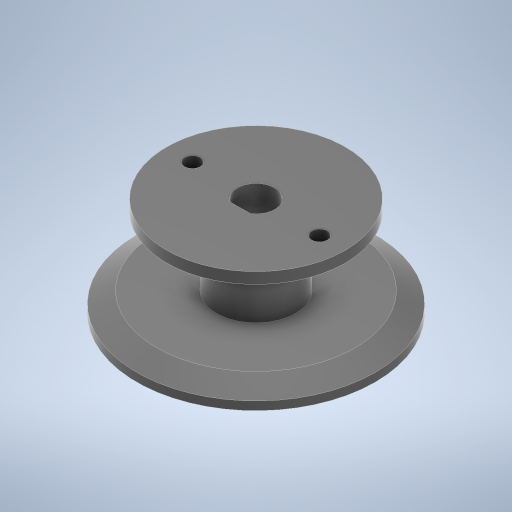
# Autodesk Inventor part: Pulley
Saved by Autodesk Inventor 2024 (Build 280153000, 153)
## iProperties
Created: 2023-12-18
Part Number: Pulley
Material: Generic
Document SubType Name: Modeling
Designer: greg
Density: 1 g/cm^3
Appearance: Smooth - Black
Author: greg
## iProperties of the stored document Pulley_3DPrint.ipt
Created: 2023-12-18
Part Number: Pulley_3DPrint
Material: Generic
Document SubType Name: Modeling
Designer: greg
Density: 1 g/cm^3
Appearance: Default
Author: greg
Autodesk Inventor part; units mm, degrees
ref_plane "YZ Plane" through (0, 0, 0) normal (1, 0, 0) x (0, 1, 0)
ref_plane "XZ Plane" through (0, 0, 0) normal (0, 1, 0) x (-1, 0, 0)
ref_plane "XY Plane" through (0, 0, 0) normal (0, 0, 1) x (1, 0, 0)
sketch "Sketch1" plane through (0, 0, 0) normal (0, 1, 0) x (-1, 0, 0)
  circle A0 centre (0, 0) radius 19.05
  dimension "d0" = 38.1
  constraints: 1 centre point, 1 coincident
  measures "d0" diameter of A0
extrude "Extrusion1" add sketch "Sketch1" along normal blind 3.175
sketch "Sketch2" plane through (0, 3.175, 0) normal (0, 1, 0) x (1, 0, 0)
  circle A0 centre (0, 0) radius 6.35
  dimension "d3" = 12.7
  constraints: 1 centre point, 1 coincident
  measures "d3" diameter of A0
extrude "Extrusion2" add sketch "Sketch2" along normal blind 6.35
sketch "Sketch3" plane through (0, 9.525, 0) normal (0, 1, 0) x (1, 0, 0)
  circle A0 centre (0, 0) radius 14.2875
  dimension "d6" = 28.575
  constraints: 1 centre point, 1 coincident
  measures "d6" diameter of A0
extrude "Extrusion3" add sketch "Sketch3" along normal blind 6.35
chamfer "Chamfer1" distance 7.9375 angle 30 1 edges at (-14.2875, 9.525, 0) measured on face at (-13.7875, 9.525, 0)
chamfer "Chamfer2" distance 3.175 angle 30 1 edges at (19.05, 3.175, 0) measured on face at (18.55, 3.175, 0)
sketch "Sketch4" plane through (0, 15.875, 0) normal (0, 1, 0) x (1, 0, 0)
  circle A0 centre (-10.16, 0) radius 1.27
  circle A1 centre (10.16, 0) radius 1.27
  circle A2 centre (0, 0) radius 6.35 projected
  dimension "d15" = 2.54
  dimension "d16" = 10.16
  dimension "d17" = 10.16
  constraints: 2 centre point, 1 equal radius
  measures "d15" diameter of A0
  measures "d16" distance of A0.centre A2.centre
  measures "d17" distance of A1.centre point (0, 0)
extrude "Extrusion4" cut sketch "Sketch4" against normal up to surface (12.7 mm away) contours A0 | A1
sketch "Sketch5" plane through (0, 15.875, 0) normal (0, 1, 0) x (1, 0, 0)
  circle A0 centre (0, 0) radius 3
  line L0 (-1.6583, -2.5) -> (1.6583, -2.5)
  point P0 (0, 3)
  dimension "d20" = 6
  dimension "d21" = 5.5
  constraints: 3 point on circle, 2 end point, 1 centre point, 1 coincident, 1 horizontal, 1 vertical alignment
  measures "d20" diameter of A0
  measures "d21" distance from line of L0 point (0, 3)
extrude "Extrusion5" cut sketch "Sketch5" against normal through all contours A0 L0 picked at (0.1141, -0.6732)
equation "\"d17\" = d16"
body "Solid1"
